Autodesk Inventor part; units mm, degrees
(part 2 of 2)
  line L664 (19.8841, -6.2623) -> (19.8841, -5.9623)
  arc A222 (19.8841, -6.2623) -> (19.8841, -7.2623) centre (19.8841, -6.7623) ccw
  arc A223 (18.2741, -5.9623) -> (18.2741, -7.5623) centre (18.2741, -6.7623) ccw
  arc A224 (18.2741, -5.9623) -> (18.2741, -7.5623) centre (18.2741, -6.7623) ccw
  line L665 (19.8841, -7.5623) -> (18.2741, -7.5623)
  line L666 (18.2741, -7.5623) -> (19.8841, -7.5623)
  line L667 (19.8841, -7.5623) -> (19.8841, -7.2623)
  circle A225 centre (18.2741, -6.7623) radius 0.5
  circle A226 centre (18.2741, -11.8423) radius 0.5
  circle A227 centre (6.8441, -19.2223) radius 0.5
  line L668 (-1.1159, -15.1823) -> (-1.1159, -16.1223)
  line L669 (-1.1159, -14.8823) -> (-1.1159, -16.4223)
  arc A228 (-1.1159, -17.4223) -> (-1.1159, -16.4223) centre (-1.1159, -16.9223) ccw
  circle A229 centre (0.4941, -16.9223) radius 0.5
  line L670 (-1.1159, -17.7223) -> (-1.1159, -18.6623)
  line L671 (-1.1159, -17.4223) -> (-1.1159, -18.9623)
  arc A230 (-1.1159, -19.9623) -> (-1.1159, -18.9623) centre (-1.1159, -19.4623) ccw
  line L672 (-1.1159, -20.2623) -> (-1.1159, -20.3323)
  arc A231 (7.3441, -20.8323) -> (6.3441, -20.8323) centre (6.8441, -20.8323) ccw
  line L673 (-1.1159, -19.9623) -> (-1.1159, -20.3323)
  arc A232 (19.8841, -8.8023) -> (19.8841, -9.8023) centre (19.8841, -9.3023) ccw
  arc A233 (19.8841, -13.8823) -> (19.8841, -14.8823) centre (19.8841, -14.3823) ccw
  arc A234 (19.8841, -18.9623) -> (19.8841, -19.9623) centre (19.8841, -19.4623) ccw
  line L674 (19.8841, -20.2623) -> (19.8841, -19.9623)
  circle A235 centre (18.2741, -19.4623) radius 0.5
  circle A236 centre (18.2741, -19.4623) radius 0.5
  circle A237 centre (9.3841, -19.2223) radius 0.5
  line L675 (-1.1159, -18.6623) -> (-1.1159, -18.9623)
  circle A238 centre (0.4941, -19.4623) radius 0.5
  circle A239 centre (0.4941, -19.4623) radius 0.5
  line L676 (-1.1159, -20.2623) -> (0.4941, -20.2623)
  line L677 (-1.1159, -19.9623) -> (-1.1159, -20.2623)
  arc A240 (-1.1159, -19.9623) -> (-1.1159, -18.9623) centre (-1.1159, -19.4623) ccw
  arc A241 (19.8841, -16.4223) -> (19.8841, -17.4223) centre (19.8841, -16.9223) ccw
  arc A242 (9.8841, -20.8323) -> (8.8841, -20.8323) centre (9.3841, -20.8323) ccw
  arc A243 (12.4241, -20.8323) -> (11.4241, -20.8323) centre (11.9241, -20.8323) ccw
  circle A244 centre (18.2741, -16.9223) radius 0.5
  circle A245 centre (18.2741, -14.3823) radius 0.5
  arc A246 (19.8841, -18.9623) -> (19.8841, -19.9623) centre (19.8841, -19.4623) ccw
  circle A247 centre (11.9241, -19.2223) radius 0.5
  line L678 (19.8841, -18.6623) -> (18.2741, -18.6623)
  line L679 (18.2741, -18.6623) -> (19.8841, -18.6623)
  arc A248 (18.2741, -18.6623) -> (18.2741, -20.2623) centre (18.2741, -19.4623) ccw
  arc A249 (18.2741, -18.6623) -> (18.2741, -20.2623) centre (18.2741, -19.4623) ccw
  line L680 (18.2741, -20.2623) -> (19.8841, -20.2623)
  line L681 (19.8841, -20.2623) -> (18.2741, -20.2623)
  line L682 (19.8841, -18.9623) -> (19.8841, -18.6623)
  arc A250 (0.4941, -20.2623) -> (0.4941, -18.6623) centre (0.4941, -19.4623) ccw
  arc A251 (0.4941, -20.2623) -> (0.4941, -18.6623) centre (0.4941, -19.4623) ccw
  line L683 (0.4941, -18.6623) -> (-1.1159, -18.6623)
  line L684 (-1.1159, -18.6623) -> (0.4941, -18.6623)
  line L685 (0.4941, -20.2623) -> (-1.1159, -20.2623)
  line L686 (-1.1159, -8.5023) -> (0.4941, -8.5023)
  line L687 (0.4941, -7.5623) -> (-1.1159, -7.5623)
  line L688 (-1.1159, -7.5623) -> (0.4941, -7.5623)
  line L689 (-1.1159, -7.2623) -> (-1.1159, -7.5623)
  circle A252 centre (0.4941, -6.7623) radius 0.5
  arc A253 (0.4941, -7.5623) -> (0.4941, -5.9623) centre (0.4941, -6.7623) ccw
  arc A254 (0.4941, -7.5623) -> (0.4941, -5.9623) centre (0.4941, -6.7623) ccw
  arc A255 (-1.1159, -7.2623) -> (-1.1159, -6.2623) centre (-1.1159, -6.7623) ccw
  line L690 (0.4941, -5.9623) -> (-1.1159, -5.9623)
  line L691 (-1.1159, -5.9623) -> (-1.1159, -6.2623)
  line L692 (-1.1159, -5.9623) -> (0.4941, -5.9623)
  line L693 (0.4941, -8.5023) -> (-1.1159, -8.5023)
  circle A256 centre (0.4941, -11.8423) radius 0.5
  arc A257 (-1.1159, -12.3423) -> (-1.1159, -11.3423) centre (-1.1159, -11.8423) ccw
  line L694 (-1.1159, -11.0423) -> (-1.1159, -11.3423)
  line L695 (-1.1159, -12.3423) -> (-1.1159, -12.6423)
  line L696 (-1.1159, -12.6423) -> (0.4941, -12.6423)
  line L697 (0.4941, -12.6423) -> (-1.1159, -12.6423)
  arc A258 (0.4941, -12.6423) -> (0.4941, -11.0423) centre (0.4941, -11.8423) ccw
  line L698 (-1.1159, -8.5023) -> (-1.1159, -8.8023)
  circle A259 centre (0.4941, -9.3023) radius 0.5
  arc A260 (-1.1159, -9.8023) -> (-1.1159, -8.8023) centre (-1.1159, -9.3023) ccw
  line L699 (-1.1159, -9.8023) -> (-1.1159, -10.1023)
  line L700 (-1.1159, -10.1023) -> (0.4941, -10.1023)
  line L701 (0.4941, -10.1023) -> (-1.1159, -10.1023)
  arc A261 (0.4941, -10.1023) -> (0.4941, -8.5023) centre (0.4941, -9.3023) ccw
  line L702 (0.4941, -11.0423) -> (-1.1159, -11.0423)
  line L703 (-1.1159, -11.0423) -> (0.4941, -11.0423)
  arc A262 (0.4941, -12.6423) -> (0.4941, -11.0423) centre (0.4941, -11.8423) ccw
  arc A263 (0.4941, -10.1023) -> (0.4941, -8.5023) centre (0.4941, -9.3023) ccw
  line L704 (-1.1159, -5.0223) -> (0.4941, -5.0223)
  line L705 (0.4941, -5.0223) -> (-1.1159, -5.0223)
  line L706 (-1.1159, -4.7223) -> (-1.1159, -5.0223)
  arc A264 (-1.1159, -4.7223) -> (-1.1159, -3.7223) centre (-1.1159, -4.2223) ccw
  line L707 (-1.1159, -3.4223) -> (-1.1159, -3.7223)
  line L708 (0.4941, -3.4223) -> (-1.1159, -3.4223)
  line L709 (-1.1159, -3.4223) -> (0.4941, -3.4223)
  circle A265 centre (0.4941, -4.2223) radius 0.5
  arc A266 (0.4941, -5.0223) -> (0.4941, -3.4223) centre (0.4941, -4.2223) ccw
  arc A267 (0.4941, -5.0223) -> (0.4941, -3.4223) centre (0.4941, -4.2223) ccw
  line L710 (18.2741, -3.4223) -> (19.8841, -3.4223)
  arc A268 (18.2741, -3.4223) -> (18.2741, -5.0223) centre (18.2741, -4.2223) ccw
  line L711 (19.8841, -5.0223) -> (18.2741, -5.0223)
  line L712 (18.2741, -5.0223) -> (19.8841, -5.0223)
  circle A269 centre (18.2741, -14.3823) radius 0.5
  arc A270 (18.2741, -3.4223) -> (18.2741, -5.0223) centre (18.2741, -4.2223) ccw
  circle A271 centre (18.2741, -11.8423) radius 0.5
  line L713 (19.8841, -11.0423) -> (18.2741, -11.0423)
  line L714 (18.2741, -11.0423) -> (19.8841, -11.0423)
  line L715 (19.8841, -11.3423) -> (19.8841, -11.0423)
  arc A272 (19.8841, -11.3423) -> (19.8841, -12.3423) centre (19.8841, -11.8423) ccw
  line L716 (18.2741, -12.6423) -> (19.8841, -12.6423)
  line L717 (19.8841, -12.6423) -> (18.2741, -12.6423)
  line L718 (19.8841, -12.6423) -> (19.8841, -12.3423)
  arc A273 (18.2741, -11.0423) -> (18.2741, -12.6423) centre (18.2741, -11.8423) ccw
  arc A274 (18.2741, -11.0423) -> (18.2741, -12.6423) centre (18.2741, -11.8423) ccw
  circle A275 centre (18.2741, -16.9223) radius 0.5
  line L719 (19.8841, -16.1223) -> (18.2741, -16.1223)
  line L720 (18.2741, -16.1223) -> (19.8841, -16.1223)
  line L721 (19.8841, -16.4223) -> (19.8841, -16.1223)
  arc A276 (19.8841, -16.4223) -> (19.8841, -17.4223) centre (19.8841, -16.9223) ccw
  arc A277 (18.2741, -16.1223) -> (18.2741, -17.7223) centre (18.2741, -16.9223) ccw
  arc A278 (18.2741, -16.1223) -> (18.2741, -17.7223) centre (18.2741, -16.9223) ccw
  line L722 (19.8841, -17.7223) -> (19.8841, -17.4223)
  line L723 (18.2741, -17.7223) -> (19.8841, -17.7223)
  line L724 (19.8841, -17.7223) -> (18.2741, -17.7223)
  circle A279 centre (11.9241, -19.2223) radius 0.5
  arc A280 (12.7241, -19.2223) -> (11.1241, -19.2223) centre (11.9241, -19.2223) ccw
  arc A281 (12.7241, -19.2223) -> (11.1241, -19.2223) centre (11.9241, -19.2223) ccw
  line L725 (12.7241, -20.8323) -> (12.7241, -19.2223)
  line L726 (12.7241, -19.2223) -> (12.7241, -20.8323)
  line L727 (12.4241, -20.8323) -> (12.7241, -20.8323)
  arc A282 (12.4241, -20.8323) -> (11.4241, -20.8323) centre (11.9241, -20.8323) ccw
  line L728 (11.1241, -20.8323) -> (11.4241, -20.8323)
  line L729 (11.1241, -20.8323) -> (11.1241, -19.2223)
  line L730 (11.1241, -19.2223) -> (11.1241, -20.8323)
  line L731 (-1.1159, -15.1823) -> (0.4941, -15.1823)
  circle A283 centre (6.8441, -19.2223) radius 0.5
  arc A284 (7.6441, -19.2223) -> (6.0441, -19.2223) centre (6.8441, -19.2223) ccw
  arc A285 (7.6441, -19.2223) -> (6.0441, -19.2223) centre (6.8441, -19.2223) ccw
  line L732 (7.6441, -20.8323) -> (7.6441, -19.2223)
  line L733 (7.6441, -19.2223) -> (7.6441, -20.8323)
  line L734 (7.3441, -20.8323) -> (7.6441, -20.8323)
  arc A286 (7.3441, -20.8323) -> (6.3441, -20.8323) centre (6.8441, -20.8323) ccw
  line L735 (6.0441, -19.2223) -> (6.0441, -20.8323)
  line L736 (6.0441, -20.8323) -> (6.0441, -19.2223)
  line L737 (6.0441, -20.8323) -> (6.3441, -20.8323)
  arc A287 (0.4941, -17.7223) -> (0.4941, -16.1223) centre (0.4941, -16.9223) ccw
  arc A288 (0.4941, -17.7223) -> (0.4941, -16.1223) centre (0.4941, -16.9223) ccw
  arc A289 (0.4941, -15.1823) -> (0.4941, -13.5823) centre (0.4941, -14.3823) ccw
  arc A290 (0.4941, -15.1823) -> (0.4941, -13.5823) centre (0.4941, -14.3823) ccw
  line L738 (0.4941, -13.5823) -> (-1.1159, -13.5823)
  line L739 (-1.1159, -13.5823) -> (0.4941, -13.5823)
  circle A291 centre (0.4941, -14.3823) radius 0.5
  line L740 (-1.1159, -13.5823) -> (-1.1159, -13.8823)
  arc A292 (-1.1159, -14.8823) -> (-1.1159, -13.8823) centre (-1.1159, -14.3823) ccw
  line L741 (-1.1159, -14.8823) -> (-1.1159, -15.1823)
  line L742 (0.4941, -15.1823) -> (-1.1159, -15.1823)
  circle A293 centre (0.4941, -16.9223) radius 0.5
  line L743 (-1.1159, -16.1223) -> (-1.1159, -16.4223)
  arc A294 (-1.1159, -17.4223) -> (-1.1159, -16.4223) centre (-1.1159, -16.9223) ccw
  line L744 (-1.1159, -17.7223) -> (0.4941, -17.7223)
  line L745 (-1.1159, -17.4223) -> (-1.1159, -17.7223)
  line L746 (-1.1159, -16.1223) -> (0.4941, -16.1223)
  line L747 (0.4941, -17.7223) -> (-1.1159, -17.7223)
  line L748 (0.4941, -16.1223) -> (-1.1159, -16.1223)
  line L749 (19.8841, 19.1377) -> (19.8841, 19.4377)
  arc A295 (19.8841, 19.1377) -> (19.8841, 18.1377) centre (19.8841, 18.6377) ccw
  line L750 (19.8841, 16.8977) -> (18.2741, 16.8977)
  line L751 (18.2741, 16.8977) -> (19.8841, 16.8977)
  line L752 (19.8841, 16.5977) -> (19.8841, 16.8977)
  circle A296 centre (18.2741, 16.0977) radius 0.5
  arc A297 (18.2741, 16.8977) -> (18.2741, 15.2977) centre (18.2741, 16.0977) ccw
  arc A298 (18.2741, 16.8977) -> (18.2741, 15.2977) centre (18.2741, 16.0977) ccw
  arc A299 (19.8841, 16.5977) -> (19.8841, 15.5977) centre (19.8841, 16.0977) ccw
  line L753 (18.2741, 15.2977) -> (19.8841, 15.2977)
  line L754 (19.8841, 15.2977) -> (18.2741, 15.2977)
  line L755 (19.8841, 15.2977) -> (19.8841, 15.5977)
  line L756 (13.0841, 31.4677) -> (13.0841, 26.4677)
  line L757 (13.0841, 31.4677) -> (13.0841, 26.4677)
  line L758 (12.7841, 31.4677) -> (12.7841, 26.4677)
  line L759 (12.9841, 30.8677) -> (12.9841, 31.4677)
  line L760 (12.7841, 26.4677) -> (13.0841, 26.4677)
  line L761 (13.3841, 30.8677) -> (12.9841, 30.8677)
  line L762 (12.7841, 31.4677) -> (13.0841, 31.4677)
  line L763 (12.9841, 31.4677) -> (13.3841, 31.4677)
  circle A300 centre (18.2741, 21.1777) radius 0.5
  arc A301 (19.8841, 21.6777) -> (19.8841, 20.6777) centre (19.8841, 21.1777) ccw
  line L764 (19.8841, 20.3777) -> (19.8841, 20.6777)
  line L765 (19.8841, 21.6777) -> (19.8841, 21.9777)
  line L766 (19.8841, 21.9777) -> (18.2741, 21.9777)
  line L767 (18.2741, 21.9777) -> (19.8841, 21.9777)
  line L768 (18.2741, 20.3777) -> (19.8841, 20.3777)
  line L769 (19.8841, 20.3777) -> (18.2741, 20.3777)
  arc A302 (18.2741, 21.9777) -> (18.2741, 20.3777) centre (18.2741, 21.1777) ccw
  arc A303 (18.2741, 21.9777) -> (18.2741, 20.3777) centre (18.2741, 21.1777) ccw
  line L770 (19.8841, 24.5177) -> (18.2741, 24.5177)
  line L771 (18.2741, 24.5177) -> (19.8841, 24.5177)
  line L772 (19.8841, 24.2177) -> (19.8841, 24.5177)
  arc A304 (18.2741, 24.5177) -> (18.2741, 22.9177) centre (18.2741, 23.7177) ccw
  arc A305 (18.2741, 24.5177) -> (18.2741, 22.9177) centre (18.2741, 23.7177) ccw
  circle A306 centre (18.2741, 23.7177) radius 0.5
  arc A307 (19.8841, 24.2177) -> (19.8841, 23.2177) centre (19.8841, 23.7177) ccw
  line L773 (18.2741, 22.9177) -> (19.8841, 22.9177)
  line L774 (19.8841, 22.9177) -> (18.2741, 22.9177)
  line L775 (19.8841, 22.9177) -> (19.8841, 23.2177)
  circle A308 centre (18.2741, 26.2577) radius 0.5
  arc A309 (19.8841, 26.7577) -> (19.8841, 25.7577) centre (19.8841, 26.2577) ccw
  line L776 (18.2741, 25.4577) -> (19.8841, 25.4577)
  line L777 (19.8841, 25.4577) -> (18.2741, 25.4577)
  line L778 (19.8841, 25.4577) -> (19.8841, 25.7577)
  line L779 (19.8841, 26.7577) -> (19.8841, 27.0577)
  arc A310 (18.2741, 27.0577) -> (18.2741, 25.4577) centre (18.2741, 26.2577) ccw
  arc A311 (18.2741, 27.0577) -> (18.2741, 25.4577) centre (18.2741, 26.2577) ccw
  line L780 (19.8841, 27.0577) -> (18.2741, 27.0577)
  line L781 (18.2741, 27.0577) -> (19.8841, 27.0577)
  circle A312 centre (18.2741, 28.7977) radius 0.5
  arc A313 (19.8841, 29.2977) -> (19.8841, 28.2977) centre (19.8841, 28.7977) ccw
  line L782 (19.8841, 27.9977) -> (19.8841, 28.2977)
  line L783 (19.8841, 29.2977) -> (19.8841, 29.5977)
  line L784 (19.8841, 29.5977) -> (18.2741, 29.5977)
  line L785 (18.2741, 29.5977) -> (19.8841, 29.5977)
  arc A314 (18.2741, 29.5977) -> (18.2741, 27.9977) centre (18.2741, 28.7977) ccw
  arc A315 (18.2741, 29.5977) -> (18.2741, 27.9977) centre (18.2741, 28.7977) ccw
  line L786 (18.2741, 27.9977) -> (19.8841, 27.9977)
  line L787 (19.8841, 27.9977) -> (18.2741, 27.9977)
  line L788 (13.3841, 31.4677) -> (13.3841, 30.8677)
  circle A316 centre (0.4941, 0.8577) radius 0.5
  arc A317 (-1.1159, 0.3577) -> (-1.1159, 1.3577) centre (-1.1159, 0.8577) ccw
  line L789 (-1.1159, 1.6577) -> (-1.1159, 1.3577)
  line L790 (-1.1159, 0.3577) -> (-1.1159, 0.0577)
  line L791 (-1.1159, 0.0577) -> (0.4941, 0.0577)
  arc A318 (0.4941, 0.0577) -> (0.4941, 1.6577) centre (0.4941, 0.8577) ccw
  arc A319 (0.4941, 0.0577) -> (0.4941, 1.6577) centre (0.4941, 0.8577) ccw
  line L792 (0.4941, 0.0577) -> (-1.1159, 0.0577)
  line L793 (0.4941, 1.6577) -> (-1.1159, 1.6577)
  line L794 (-1.1159, 1.6577) -> (0.4941, 1.6577)
  line L795 (-1.1159, 2.8977) -> (-1.1159, 2.5977)
  circle A320 centre (0.4941, 3.3977) radius 0.5
  arc A321 (-1.1159, 2.8977) -> (-1.1159, 3.8977) centre (-1.1159, 3.3977) ccw
  line L796 (-1.1159, 4.1977) -> (-1.1159, 3.8977)
  circle A322 centre (0.4941, 5.9377) radius 0.5
  arc A323 (-1.1159, 5.4377) -> (-1.1159, 6.4377) centre (-1.1159, 5.9377) ccw
  line L797 (-1.1159, 6.7377) -> (-1.1159, 6.4377)
  line L798 (-1.1159, 5.4377) -> (-1.1159, 5.1377)
  line L799 (-1.1159, 5.1377) -> (0.4941, 5.1377)
  line L800 (0.4941, 5.1377) -> (-1.1159, 5.1377)
  arc A324 (0.4941, 5.1377) -> (0.4941, 6.7377) centre (0.4941, 5.9377) ccw
  arc A325 (0.4941, 5.1377) -> (0.4941, 6.7377) centre (0.4941, 5.9377) ccw
  line L801 (0.4941, 6.7377) -> (-1.1159, 6.7377)
  line L802 (-1.1159, 6.7377) -> (0.4941, 6.7377)
  line L803 (-1.1159, 14.3577) -> (-1.1159, 14.0577)
  circle A326 centre (0.4941, 13.5577) radius 0.5
  line L804 (-1.1159, 13.0577) -> (-1.1159, 12.7577)
  line L805 (0.4941, 4.1977) -> (-1.1159, 4.1977)
  line L806 (-1.1159, 4.1977) -> (0.4941, 4.1977)
  line L807 (0.4941, 2.5977) -> (-1.1159, 2.5977)
  arc A327 (0.4941, 2.5977) -> (0.4941, 4.1977) centre (0.4941, 3.3977) ccw
  arc A328 (0.4941, 2.5977) -> (0.4941, 4.1977) centre (0.4941, 3.3977) ccw
  line L808 (-1.1159, 2.5977) -> (0.4941, 2.5977)
  arc A329 (-1.1159, 13.0577) -> (-1.1159, 14.0577) centre (-1.1159, 13.5577) ccw
  circle A330 centre (0.4941, 11.0177) radius 0.5
  arc A331 (-1.1159, 10.5177) -> (-1.1159, 11.5177) centre (-1.1159, 11.0177) ccw
  line L809 (-1.1159, 11.8177) -> (-1.1159, 11.5177)
  line L810 (-1.1159, 10.5177) -> (-1.1159, 10.2177)
  line L811 (-1.1159, 10.2177) -> (0.4941, 10.2177)
  line L812 (0.4941, 10.2177) -> (-1.1159, 10.2177)
  arc A332 (0.4941, 10.2177) -> (0.4941, 11.8177) centre (0.4941, 11.0177) ccw
  arc A333 (0.4941, 10.2177) -> (0.4941, 11.8177) centre (0.4941, 11.0177) ccw
  line L813 (-1.1159, 11.8177) -> (0.4941, 11.8177)
  line L814 (0.4941, 11.8177) -> (-1.1159, 11.8177)
  arc A334 (0.4941, 12.7577) -> (0.4941, 14.3577) centre (0.4941, 13.5577) ccw
  arc A335 (0.4941, 12.7577) -> (0.4941, 14.3577) centre (0.4941, 13.5577) ccw
  line L815 (0.4941, 14.3577) -> (-1.1159, 14.3577)
  line L816 (-1.1159, 14.3577) -> (0.4941, 14.3577)
  line L817 (0.4941, 12.7577) -> (-1.1159, 12.7577)
  line L818 (-1.1159, 12.7577) -> (0.4941, 12.7577)
  line L819 (19.8841, -3.4223) -> (18.2741, -3.4223)
  line L820 (19.8841, -3.7223) -> (19.8841, -3.4223)
  arc A336 (19.8841, -3.7223) -> (19.8841, -4.7223) centre (19.8841, -4.2223) ccw
  line L821 (19.8841, -5.0223) -> (19.8841, -4.7223)
  circle A337 centre (18.2741, -4.2223) radius 0.5
  arc A338 (19.8841, -13.8823) -> (19.8841, -14.8823) centre (19.8841, -14.3823) ccw
  line L822 (19.8841, -15.1823) -> (19.8841, -14.8823)
  line L823 (19.8841, -13.8823) -> (19.8841, -13.5823)
  line L824 (19.8841, -13.5823) -> (18.2741, -13.5823)
  line L825 (18.2741, -13.5823) -> (19.8841, -13.5823)
  circle A339 centre (9.3841, -19.2223) radius 0.5
  arc A340 (18.2741, -13.5823) -> (18.2741, -15.1823) centre (18.2741, -14.3823) ccw
  arc A341 (18.2741, -13.5823) -> (18.2741, -15.1823) centre (18.2741, -14.3823) ccw
  line L826 (18.2741, -15.1823) -> (19.8841, -15.1823)
  line L827 (19.8841, -15.1823) -> (18.2741, -15.1823)
  arc A342 (10.1841, -19.2223) -> (8.5841, -19.2223) centre (9.3841, -19.2223) ccw
  arc A343 (10.1841, -19.2223) -> (8.5841, -19.2223) centre (9.3841, -19.2223) ccw
  line L828 (8.5841, -19.2223) -> (8.5841, -20.8323)
  line L829 (8.5841, -20.8323) -> (8.5841, -19.2223)
  line L830 (10.1841, -20.8323) -> (10.1841, -19.2223)
  line L831 (10.1841, -19.2223) -> (10.1841, -20.8323)
  line L832 (9.8841, -20.8323) -> (10.1841, -20.8323)
  line L833 (8.5841, -20.8323) -> (8.8841, -20.8323)
  arc A344 (9.8841, -20.8323) -> (8.8841, -20.8323) centre (9.3841, -20.8323) ccw
  line L834 (57.2841, 13.4177) -> (56.4841, 13.4177)
  line L835 (56.4841, 13.4177) -> (57.2841, 13.4177)
  line L836 (57.2841, 13.4177) -> (57.2841, 13.9177)
  line L837 (57.2841, 13.9177) -> (56.4841, 13.9177)
  line L838 (57.2841, 13.9177) -> (57.2841, 13.4177)
  line L839 (56.4841, 13.9177) -> (57.2841, 13.9177)
  line L840 (56.4841, 13.9177) -> (56.4841, 13.4177)
  line L841 (56.4841, 13.4177) -> (56.4841, 13.9177)
  line L842 (56.4841, 8.9177) -> (57.2841, 8.9177)
  line L843 (56.4841, 8.4177) -> (56.4841, 8.9177)
  line L844 (57.2841, 8.4177) -> (56.4841, 8.4177)
  line L845 (57.2841, 8.9177) -> (57.2841, 8.4177)
  circle A345 centre (54.3841, 11.1677) radius 1.9
  circle A346 centre (54.3841, 11.1677) radius 1.9
  line L846 (57.2841, 8.9177) -> (56.4841, 8.9177)
  line L847 (56.4841, 8.9177) -> (56.4841, 8.4177)
  line L848 (57.2841, 8.4177) -> (57.2841, 8.9177)
  line L849 (56.4841, 8.4177) -> (57.2841, 8.4177)
  line L850 (52.2841, 8.9177) -> (52.2841, 8.4177)
  line L851 (52.2841, 8.4177) -> (51.4841, 8.4177)
  line L852 (51.4841, 8.4177) -> (51.4841, 8.9177)
  line L853 (51.4841, 8.9177) -> (52.2841, 8.9177)
  line L854 (52.2841, 8.9177) -> (51.4841, 8.9177)
  line L855 (52.2841, 8.4177) -> (52.2841, 8.9177)
  line L856 (51.4841, 8.9177) -> (51.4841, 8.4177)
  line L857 (51.4841, 8.4177) -> (52.2841, 8.4177)
  line L858 (52.2841, 13.4177) -> (51.4841, 13.4177)
  line L859 (51.4841, 13.4177) -> (51.4841, 13.9177)
  line L860 (51.4841, 13.9177) -> (52.2841, 13.9177)
  line L861 (52.2841, 13.4177) -> (52.2841, 13.9177)
  line L862 (52.2841, 13.9177) -> (52.2841, 13.4177)
  line L863 (52.2841, 13.9177) -> (51.4841, 13.9177)
  line L864 (51.4841, 13.9177) -> (51.4841, 13.4177)
  line L865 (51.4841, 13.4177) -> (52.2841, 13.4177)
  arc A347 (59.9841, 13.3217) -> (59.9841, 9.0136) centre (54.3841, 11.1677) ccw
  line L866 (59.9841, 9.0136) -> (59.9841, 13.3217)
  circle A348 centre (54.3841, 11.1677) radius 4.5
  circle A349 centre (54.3841, 11.1677) radius 4.5
  line L867 (59.9841, 9.0136) -> (59.9841, 13.3217)
  arc A350 (59.9841, 13.3217) -> (59.9841, 9.0136) centre (54.3841, 11.1677) ccw
  line L868 (66.6341, 18.2677) -> (66.6341, 19.0677)
  line L869 (66.6341, 19.0677) -> (66.6341, 18.2677)
  line L870 (66.6341, 18.2677) -> (67.1341, 18.2677)
  line L871 (67.1341, 18.2677) -> (67.1341, 19.0677)
  line L872 (67.1341, 18.2677) -> (66.6341, 18.2677)
  line L873 (67.1341, 19.0677) -> (67.1341, 18.2677)
  line L874 (67.1341, 19.0677) -> (66.6341, 19.0677)
  line L875 (66.6341, 19.0677) -> (67.1341, 19.0677)
  line L876 (62.1341, 19.0677) -> (62.1341, 18.2677)
  line L877 (61.6341, 19.0677) -> (62.1341, 19.0677)
  line L878 (61.6341, 18.2677) -> (61.6341, 19.0677)
  line L879 (62.1341, 18.2677) -> (61.6341, 18.2677)
  circle A351 centre (64.3841, 21.1677) radius 1.9
  circle A352 centre (64.3841, 21.1677) radius 1.9
  line L880 (62.1341, 18.2677) -> (62.1341, 19.0677)
  line L881 (62.1341, 19.0677) -> (61.6341, 19.0677)
  line L882 (61.6341, 18.2677) -> (62.1341, 18.2677)
  line L883 (61.6341, 19.0677) -> (61.6341, 18.2677)
  line L884 (62.1341, 23.2677) -> (61.6341, 23.2677)
  line L885 (61.6341, 23.2677) -> (61.6341, 24.0677)
  line L886 (61.6341, 24.0677) -> (62.1341, 24.0677)
  line L887 (62.1341, 24.0677) -> (62.1341, 23.2677)
  line L888 (62.1341, 23.2677) -> (62.1341, 24.0677)
  line L889 (61.6341, 23.2677) -> (62.1341, 23.2677)
  line L890 (62.1341, 24.0677) -> (61.6341, 24.0677)
  line L891 (61.6341, 24.0677) -> (61.6341, 23.2677)
  line L892 (66.6341, 23.2677) -> (66.6341, 24.0677)
  line L893 (66.6341, 24.0677) -> (67.1341, 24.0677)
  line L894 (67.1341, 24.0677) -> (67.1341, 23.2677)
  line L895 (66.6341, 23.2677) -> (67.1341, 23.2677)
  line L896 (67.1341, 23.2677) -> (66.6341, 23.2677)
  line L897 (67.1341, 23.2677) -> (67.1341, 24.0677)
  line L898 (67.1341, 24.0677) -> (66.6341, 24.0677)
  line L899 (66.6341, 24.0677) -> (66.6341, 23.2677)
  arc A353 (66.5382, 15.5677) -> (62.2301, 15.5677) centre (64.3841, 21.1677) ccw
  line L900 (62.2301, 15.5677) -> (66.5382, 15.5677)
  circle A354 centre (64.3841, 21.1677) radius 4.5
  circle A355 centre (64.3841, 21.1677) radius 4.5
  line L901 (62.2301, 15.5677) -> (66.5382, 15.5677)
  arc A356 (66.5382, 15.5677) -> (62.2301, 15.5677) centre (64.3841, 21.1677) ccw
  line L902 (62.1341, 4.0677) -> (62.1341, 3.2677)
  line L903 (62.1341, 3.2677) -> (62.1341, 4.0677)
  line L904 (62.1341, 4.0677) -> (61.6341, 4.0677)
  line L905 (61.6341, 4.0677) -> (61.6341, 3.2677)
  line L906 (61.6341, 4.0677) -> (62.1341, 4.0677)
  line L907 (61.6341, 3.2677) -> (61.6341, 4.0677)
  line L908 (61.6341, 3.2677) -> (62.1341, 3.2677)
  line L909 (62.1341, 3.2677) -> (61.6341, 3.2677)
  line L910 (66.6341, 3.2677) -> (66.6341, 4.0677)
  line L911 (67.1341, 3.2677) -> (66.6341, 3.2677)
  line L912 (67.1341, 4.0677) -> (67.1341, 3.2677)
  line L913 (66.6341, 4.0677) -> (67.1341, 4.0677)
  circle A357 centre (64.3841, 1.1677) radius 1.9
  circle A358 centre (64.3841, 1.1677) radius 1.9
  line L914 (66.6341, 4.0677) -> (66.6341, 3.2677)
  line L915 (66.6341, 3.2677) -> (67.1341, 3.2677)
  line L916 (67.1341, 4.0677) -> (66.6341, 4.0677)
  line L917 (67.1341, 3.2677) -> (67.1341, 4.0677)
  line L918 (66.6341, -0.9323) -> (67.1341, -0.9323)
  line L919 (67.1341, -0.9323) -> (67.1341, -1.7323)
  line L920 (67.1341, -1.7323) -> (66.6341, -1.7323)
  line L921 (66.6341, -1.7323) -> (66.6341, -0.9323)
  line L922 (66.6341, -0.9323) -> (66.6341, -1.7323)
  line L923 (67.1341, -0.9323) -> (66.6341, -0.9323)
  line L924 (66.6341, -1.7323) -> (67.1341, -1.7323)
  line L925 (67.1341, -1.7323) -> (67.1341, -0.9323)
  line L926 (62.1341, -0.9323) -> (62.1341, -1.7323)
  line L927 (62.1341, -1.7323) -> (61.6341, -1.7323)
  line L928 (61.6341, -1.7323) -> (61.6341, -0.9323)
  line L929 (62.1341, -0.9323) -> (61.6341, -0.9323)
  line L930 (61.6341, -0.9323) -> (62.1341, -0.9323)
  line L931 (61.6341, -0.9323) -> (61.6341, -1.7323)
  line L932 (61.6341, -1.7323) -> (62.1341, -1.7323)
  line L933 (62.1341, -1.7323) -> (62.1341, -0.9323)
  arc A359 (62.2301, 6.7677) -> (66.5382, 6.7677) centre (64.3841, 1.1677) ccw
  line L934 (66.5382, 6.7677) -> (62.2301, 6.7677)
  circle A360 centre (64.3841, 1.1677) radius 4.5
  circle A361 centre (64.3841, 1.1677) radius 4.5
  line L935 (66.5382, 6.7677) -> (62.2301, 6.7677)
  arc A362 (62.2301, 6.7677) -> (66.5382, 6.7677) centre (64.3841, 1.1677) ccw
  line L936 (71.4841, 8.9177) -> (72.2841, 8.9177)
  line L937 (72.2841, 8.9177) -> (71.4841, 8.9177)
  line L938 (71.4841, 8.9177) -> (71.4841, 8.4177)
  line L939 (71.4841, 8.4177) -> (72.2841, 8.4177)
  line L940 (71.4841, 8.4177) -> (71.4841, 8.9177)
  line L941 (72.2841, 8.4177) -> (71.4841, 8.4177)
  line L942 (72.2841, 8.4177) -> (72.2841, 8.9177)
  line L943 (72.2841, 8.9177) -> (72.2841, 8.4177)
  line L944 (72.2841, 13.4177) -> (71.4841, 13.4177)
  line L945 (72.2841, 13.9177) -> (72.2841, 13.4177)
  line L946 (71.4841, 13.9177) -> (72.2841, 13.9177)
  line L947 (71.4841, 13.4177) -> (71.4841, 13.9177)
  circle A363 centre (74.3841, 11.1677) radius 1.9
  circle A364 centre (74.3841, 11.1677) radius 1.9
  line L948 (71.4841, 13.4177) -> (72.2841, 13.4177)
  line L949 (72.2841, 13.4177) -> (72.2841, 13.9177)
  line L950 (71.4841, 13.9177) -> (71.4841, 13.4177)
  line L951 (72.2841, 13.9177) -> (71.4841, 13.9177)
  line L952 (76.4841, 13.4177) -> (76.4841, 13.9177)
  line L953 (76.4841, 13.9177) -> (77.2841, 13.9177)
  line L954 (77.2841, 13.9177) -> (77.2841, 13.4177)
  line L955 (77.2841, 13.4177) -> (76.4841, 13.4177)
  line L956 (76.4841, 13.4177) -> (77.2841, 13.4177)
  line L957 (76.4841, 13.9177) -> (76.4841, 13.4177)
  line L958 (77.2841, 13.4177) -> (77.2841, 13.9177)
  line L959 (77.2841, 13.9177) -> (76.4841, 13.9177)
  line L960 (76.4841, 8.9177) -> (77.2841, 8.9177)
  line L961 (77.2841, 8.9177) -> (77.2841, 8.4177)
  line L962 (77.2841, 8.4177) -> (76.4841, 8.4177)
  line L963 (76.4841, 8.9177) -> (76.4841, 8.4177)
  line L964 (76.4841, 8.4177) -> (76.4841, 8.9177)
  line L965 (76.4841, 8.4177) -> (77.2841, 8.4177)
  line L966 (77.2841, 8.4177) -> (77.2841, 8.9177)
  line L967 (77.2841, 8.9177) -> (76.4841, 8.9177)
  arc A365 (68.7841, 9.0136) -> (68.7841, 13.3217) centre (74.3841, 11.1677) ccw
  line L968 (68.7841, 13.3217) -> (68.7841, 9.0136)
  circle A366 centre (74.3841, 11.1677) radius 4.5
  circle A367 centre (74.3841, 11.1677) radius 4.5
  line L969 (68.7841, 13.3217) -> (68.7841, 9.0136)
  arc A368 (68.7841, 9.0136) -> (68.7841, 13.3217) centre (74.3841, 11.1677) ccw
  line L970 (-43.3659, 18.2677) -> (-43.3659, 19.0677)
  line L971 (-43.3659, 19.0677) -> (-43.3659, 18.2677)
  line L972 (-43.3659, 18.2677) -> (-42.8659, 18.2677)
  line L973 (-42.8659, 18.2677) -> (-42.8659, 19.0677)
  line L974 (-42.8659, 18.2677) -> (-43.3659, 18.2677)
  line L975 (-42.8659, 19.0677) -> (-42.8659, 18.2677)
  line L976 (-42.8659, 19.0677) -> (-43.3659, 19.0677)
  line L977 (-43.3659, 19.0677) -> (-42.8659, 19.0677)
  line L978 (-47.8659, 19.0677) -> (-47.8659, 18.2677)
  line L979 (-48.3659, 19.0677) -> (-47.8659, 19.0677)
  line L980 (-48.3659, 18.2677) -> (-48.3659, 19.0677)
  line L981 (-47.8659, 18.2677) -> (-48.3659, 18.2677)
  circle A369 centre (-45.6159, 21.1677) radius 1.9
  circle A370 centre (-45.6159, 21.1677) radius 1.9
  line L982 (-47.8659, 18.2677) -> (-47.8659, 19.0677)
  line L983 (-47.8659, 19.0677) -> (-48.3659, 19.0677)
  line L984 (-48.3659, 18.2677) -> (-47.8659, 18.2677)
  line L985 (-48.3659, 19.0677) -> (-48.3659, 18.2677)
  line L986 (-47.8659, 23.2677) -> (-48.3659, 23.2677)
  line L987 (-48.3659, 23.2677) -> (-48.3659, 24.0677)
  line L988 (-48.3659, 24.0677) -> (-47.8659, 24.0677)
  line L989 (-47.8659, 24.0677) -> (-47.8659, 23.2677)
  line L990 (-47.8659, 23.2677) -> (-47.8659, 24.0677)
  line L991 (-48.3659, 23.2677) -> (-47.8659, 23.2677)
  line L992 (-47.8659, 24.0677) -> (-48.3659, 24.0677)
  line L993 (-48.3659, 24.0677) -> (-48.3659, 23.2677)
  line L994 (-43.3659, 23.2677) -> (-43.3659, 24.0677)
  line L995 (-43.3659, 24.0677) -> (-42.8659, 24.0677)
  line L996 (-42.8659, 24.0677) -> (-42.8659, 23.2677)
  line L997 (-43.3659, 23.2677) -> (-42.8659, 23.2677)
  line L998 (-42.8659, 23.2677) -> (-43.3659, 23.2677)
  line L999 (-42.8659, 23.2677) -> (-42.8659, 24.0677)
  line L1000 (-42.8659, 24.0677) -> (-43.3659, 24.0677)
  line L1001 (-43.3659, 24.0677) -> (-43.3659, 23.2677)
  line L1002 (-47.7699, 15.5677) -> (-43.4618, 15.5677)
  circle A371 centre (-45.6159, 21.1677) radius 4.5
  circle A372 centre (-45.6159, 21.1677) radius 4.5
  line L1003 (-47.7699, 15.5677) -> (-43.4618, 15.5677)
  arc A373 (-43.4618, 15.5677) -> (-47.7699, 15.5677) centre (-45.6159, 21.1677) ccw
  line L1004 (-47.8659, 4.0677) -> (-47.8659, 3.2677)
  line L1005 (-47.8659, 3.2677) -> (-47.8659, 4.0677)
  line L1006 (-47.8659, 4.0677) -> (-48.3659, 4.0677)
  line L1007 (-48.3659, 4.0677) -> (-48.3659, 3.2677)
  line L1008 (-48.3659, 4.0677) -> (-47.8659, 4.0677)
  line L1009 (-48.3659, 3.2677) -> (-48.3659, 4.0677)
  line L1010 (-48.3659, 3.2677) -> (-47.8659, 3.2677)
  line L1011 (-47.8659, 3.2677) -> (-48.3659, 3.2677)
  line L1012 (-43.3659, 3.2677) -> (-43.3659, 4.0677)
  line L1013 (-42.8659, 3.2677) -> (-43.3659, 3.2677)
  line L1014 (-42.8659, 4.0677) -> (-42.8659, 3.2677)
  line L1015 (-43.3659, 4.0677) -> (-42.8659, 4.0677)
  circle A374 centre (-45.6159, 1.1677) radius 1.9
  circle A375 centre (-45.6159, 1.1677) radius 1.9
  line L1016 (-43.3659, 4.0677) -> (-43.3659, 3.2677)
  line L1017 (-43.3659, 3.2677) -> (-42.8659, 3.2677)
  line L1018 (-42.8659, 4.0677) -> (-43.3659, 4.0677)
  line L1019 (-42.8659, 3.2677) -> (-42.8659, 4.0677)
  line L1020 (-43.3659, -0.9323) -> (-42.8659, -0.9323)
  line L1021 (-42.8659, -0.9323) -> (-42.8659, -1.7323)
  line L1022 (-42.8659, -1.7323) -> (-43.3659, -1.7323)
  line L1023 (-43.3659, -1.7323) -> (-43.3659, -0.9323)
  line L1024 (-43.3659, -0.9323) -> (-43.3659, -1.7323)
  line L1025 (-42.8659, -0.9323) -> (-43.3659, -0.9323)
  line L1026 (-43.3659, -1.7323) -> (-42.8659, -1.7323)
  line L1027 (-42.8659, -1.7323) -> (-42.8659, -0.9323)
  line L1028 (-47.8659, -0.9323) -> (-47.8659, -1.7323)
  line L1029 (-47.8659, -1.7323) -> (-48.3659, -1.7323)
  line L1030 (-48.3659, -1.7323) -> (-48.3659, -0.9323)
  line L1031 (-47.8659, -0.9323) -> (-48.3659, -0.9323)
  line L1032 (-48.3659, -0.9323) -> (-47.8659, -0.9323)
  line L1033 (-48.3659, -0.9323) -> (-48.3659, -1.7323)
  line L1034 (-48.3659, -1.7323) -> (-47.8659, -1.7323)
  line L1035 (-47.8659, -1.7323) -> (-47.8659, -0.9323)
  arc A376 (-47.7699, 6.7677) -> (-43.4618, 6.7677) centre (-45.6159, 1.1677) ccw
  line L1036 (-43.4618, 6.7677) -> (-47.7699, 6.7677)
  circle A377 centre (-45.6159, 1.1677) radius 4.5
  circle A378 centre (-45.6159, 1.1677) radius 4.5
  line L1037 (-43.4618, 6.7677) -> (-47.7699, 6.7677)
  arc A379 (-47.7699, 6.7677) -> (-43.4618, 6.7677) centre (-45.6159, 1.1677) ccw
  line L1038 (-38.5159, 8.9177) -> (-37.7159, 8.9177)
  line L1039 (-37.7159, 8.9177) -> (-38.5159, 8.9177)
  line L1040 (-38.5159, 8.9177) -> (-38.5159, 8.4177)
  line L1041 (-38.5159, 8.4177) -> (-37.7159, 8.4177)
  line L1042 (-38.5159, 8.4177) -> (-38.5159, 8.9177)
  line L1043 (-37.7159, 8.4177) -> (-38.5159, 8.4177)
  line L1044 (-37.7159, 8.4177) -> (-37.7159, 8.9177)
  line L1045 (-37.7159, 8.9177) -> (-37.7159, 8.4177)
  line L1046 (-37.7159, 13.4177) -> (-38.5159, 13.4177)
  line L1047 (-37.7159, 13.9177) -> (-37.7159, 13.4177)
  line L1048 (-38.5159, 13.9177) -> (-37.7159, 13.9177)
  line L1049 (-38.5159, 13.4177) -> (-38.5159, 13.9177)
  circle A380 centre (-35.6159, 11.1677) radius 1.9
  circle A381 centre (-35.6159, 11.1677) radius 1.9
  line L1050 (-38.5159, 13.4177) -> (-37.7159, 13.4177)
  line L1051 (-37.7159, 13.4177) -> (-37.7159, 13.9177)
  line L1052 (-38.5159, 13.9177) -> (-38.5159, 13.4177)
  line L1053 (-37.7159, 13.9177) -> (-38.5159, 13.9177)
  line L1054 (-33.5159, 13.4177) -> (-33.5159, 13.9177)
  line L1055 (-33.5159, 13.9177) -> (-32.7159, 13.9177)
  line L1056 (-32.7159, 13.9177) -> (-32.7159, 13.4177)
  line L1057 (-32.7159, 13.4177) -> (-33.5159, 13.4177)
  line L1058 (-33.5159, 13.4177) -> (-32.7159, 13.4177)
  line L1059 (-33.5159, 13.9177) -> (-33.5159, 13.4177)
  line L1060 (-32.7159, 13.4177) -> (-32.7159, 13.9177)
  line L1061 (-32.7159, 13.9177) -> (-33.5159, 13.9177)
  line L1062 (-33.5159, 8.9177) -> (-32.7159, 8.9177)
  line L1063 (-32.7159, 8.9177) -> (-32.7159, 8.4177)
  line L1064 (-32.7159, 8.4177) -> (-33.5159, 8.4177)
  line L1065 (-33.5159, 8.9177) -> (-33.5159, 8.4177)
  line L1066 (-33.5159, 8.4177) -> (-33.5159, 8.9177)
  line L1067 (-33.5159, 8.4177) -> (-32.7159, 8.4177)
  line L1068 (-32.7159, 8.4177) -> (-32.7159, 8.9177)
  line L1069 (-32.7159, 8.9177) -> (-33.5159, 8.9177)
  arc A382 (-41.2159, 9.0136) -> (-41.2159, 13.3217) centre (-35.6159, 11.1677) ccw
  line L1070 (-41.2159, 13.3217) -> (-41.2159, 9.0136)
  circle A383 centre (-35.6159, 11.1677) radius 4.5
  circle A384 centre (-35.6159, 11.1677) radius 4.5
  line L1071 (-41.2159, 13.3217) -> (-41.2159, 9.0136)
  arc A385 (-41.2159, 9.0136) -> (-41.2159, 13.3217) centre (-35.6159, 11.1677) ccw
  line L1072 (-52.7159, 13.4177) -> (-53.5159, 13.4177)
  line L1073 (-53.5159, 13.4177) -> (-52.7159, 13.4177)
  line L1074 (-52.7159, 13.4177) -> (-52.7159, 13.9177)
  line L1075 (-52.7159, 13.9177) -> (-53.5159, 13.9177)
  line L1076 (-52.7159, 13.9177) -> (-52.7159, 13.4177)
  line L1077 (-53.5159, 13.9177) -> (-52.7159, 13.9177)
  line L1078 (-53.5159, 13.9177) -> (-53.5159, 13.4177)
  line L1079 (-53.5159, 13.4177) -> (-53.5159, 13.9177)
  line L1080 (-53.5159, 8.9177) -> (-52.7159, 8.9177)
  line L1081 (-53.5159, 8.4177) -> (-53.5159, 8.9177)
  line L1082 (-52.7159, 8.4177) -> (-53.5159, 8.4177)
  line L1083 (-52.7159, 8.9177) -> (-52.7159, 8.4177)
  circle A386 centre (-55.6159, 11.1677) radius 1.9
  circle A387 centre (-55.6159, 11.1677) radius 1.9
  line L1084 (-52.7159, 8.9177) -> (-53.5159, 8.9177)
  line L1085 (-53.5159, 8.9177) -> (-53.5159, 8.4177)
  line L1086 (-52.7159, 8.4177) -> (-52.7159, 8.9177)
  line L1087 (-53.5159, 8.4177) -> (-52.7159, 8.4177)
  line L1088 (-57.7159, 8.9177) -> (-57.7159, 8.4177)
  line L1089 (-57.7159, 8.4177) -> (-58.5159, 8.4177)
  line L1090 (-58.5159, 8.4177) -> (-58.5159, 8.9177)
  line L1091 (-58.5159, 8.9177) -> (-57.7159, 8.9177)
  line L1092 (-57.7159, 8.9177) -> (-58.5159, 8.9177)
  line L1093 (-57.7159, 8.4177) -> (-57.7159, 8.9177)
  line L1094 (-58.5159, 8.9177) -> (-58.5159, 8.4177)
  line L1095 (-58.5159, 8.4177) -> (-57.7159, 8.4177)
  line L1096 (-57.7159, 13.4177) -> (-58.5159, 13.4177)
  line L1097 (-58.5159, 13.4177) -> (-58.5159, 13.9177)
  line L1098 (-58.5159, 13.9177) -> (-57.7159, 13.9177)
  line L1099 (-57.7159, 13.4177) -> (-57.7159, 13.9177)
  line L1100 (-57.7159, 13.9177) -> (-57.7159, 13.4177)
  line L1101 (-57.7159, 13.9177) -> (-58.5159, 13.9177)
  line L1102 (-58.5159, 13.9177) -> (-58.5159, 13.4177)
  line L1103 (-58.5159, 13.4177) -> (-57.7159, 13.4177)
  arc A388 (-50.0159, 13.3217) -> (-50.0159, 9.0136) centre (-55.6159, 11.1677) ccw
  line L1104 (-50.0159, 9.0136) -> (-50.0159, 13.3217)
  circle A389 centre (-55.6159, 11.1677) radius 4.5
  circle A390 centre (-55.6159, 11.1677) radius 4.5
  line L1105 (-50.0159, 9.0136) -> (-50.0159, 13.3217)
  arc A391 (-50.0159, 13.3217) -> (-50.0159, 9.0136) centre (-55.6159, 11.1677) ccw
  point P0 (37.3841, -10.6323)
  point P1 (-18.6159, -10.6323)
  dimension "d2" = 150
  constraints: 2204 end point, 392 centre point, 392 point on circle, 6 other
  measures "d2" distance of L2.start L36.start
sketch "Náčrt2" plane through (0, 0, 0) normal (0, 0, 1) x (1, 0, 0)
  line L0 (-66.6159, 31.6677) -> (85.3841, 31.6677)
  line L1 (85.3841, 31.6677) -> (85.3841, -29.3323)
  line L2 (85.3841, -29.3323) -> (-66.6159, -29.3323)
  line L3 (-66.6159, -29.3323) -> (-66.6159, 31.6677)
  line L4 (84.3841, 31.1677) -> (-65.6159, 31.1677) projected
  line L5 (-65.6159, 31.1677) -> (-65.6159, -28.8323) projected
  line L6 (-65.6159, -28.8323) -> (84.3841, -28.8323) projected
  line L7 (84.3841, -28.8323) -> (84.3841, 31.1677) projected
  arc A0 (-43.4618, 15.5677) -> (-47.7699, 15.5677) centre (-45.6159, 21.1677) ccw projected
  line L8 (-47.7699, 15.5677) -> (-43.4618, 15.5677) projected
  line L9 (-50.0159, 9.0136) -> (-50.0159, 13.3217) projected
  arc A1 (-50.0159, 13.3217) -> (-50.0159, 9.0136) centre (-55.6159, 11.1677) ccw projected
  line L10 (-43.4618, 6.7677) -> (-47.7699, 6.7677) projected
  arc A2 (-47.7699, 6.7677) -> (-43.4618, 6.7677) centre (-45.6159, 1.1677) ccw projected
  line L11 (-41.2159, 13.3217) -> (-41.2159, 9.0136) projected
  arc A3 (-41.2159, 9.0136) -> (-41.2159, 13.3217) centre (-35.6159, 11.1677) ccw projected
  circle A4 centre (-18.6159, -10.6323) radius 12 projected
  circle A5 centre (37.3841, -10.6323) radius 12 projected
  arc A6 (59.9841, 13.3217) -> (59.9841, 9.0136) centre (54.3841, 11.1677) ccw projected
  line L12 (59.9841, 9.0136) -> (59.9841, 13.3217) projected
  arc A7 (66.5382, 15.5677) -> (62.2301, 15.5677) centre (64.3841, 21.1677) ccw projected
  line L13 (62.2301, 15.5677) -> (66.5382, 15.5677) projected
  line L14 (68.7841, 13.3217) -> (68.7841, 9.0136) projected
  arc A8 (68.7841, 9.0136) -> (68.7841, 13.3217) centre (74.3841, 11.1677) ccw projected
  line L15 (66.5382, 6.7677) -> (62.2301, 6.7677) projected
  arc A9 (62.2301, 6.7677) -> (66.5382, 6.7677) centre (64.3841, 1.1677) ccw projected
  point P0 (0, 0)
  dimension "d5" = 0.5
  dimension "d6" = 0.5
  dimension "d7" = 1
  dimension "d8" = 1
  constraints: 8 end point, 2 parallel, 1 horizontal, 1 perpendicular
  measures "d5" distance between parallel lines of L4 L0
  measures "d6" distance between parallel lines of L6 L2
  measures "d7" distance between parallel lines of L5 L3
  measures "d8" distance between parallel lines of L7 L1
extrude "Vysunutí1" add sketch "Náčrt2" along normal blind 10 contours L0 L1 L2 L3 | L7 L6 L5 L4 | L8 A0 | A1 L9 | A2 L10 | A3 L11 | A4 | A5 | L12 A6 | L13 A7 | A8 L14 | A9 L15
sketch "Náčrt3" plane through (0, 0, 0) normal (0, 0, -1) x (-1, 0, 0)
  arc A0 (-62.2301, 15.5677) -> (-66.5382, 15.5677) centre (-64.3841, 21.1677) ccw projected
  line L0 (-62.2301, 15.5677) -> (-66.5382, 15.5677) projected
  arc A1 (-68.7841, 13.3217) -> (-68.7841, 9.0136) centre (-74.3841, 11.1677) ccw projected
  line L1 (-68.7841, 13.3217) -> (-68.7841, 9.0136) projected
  line L2 (-66.5382, 6.7677) -> (-62.2301, 6.7677) projected
  arc A2 (-66.5382, 6.7677) -> (-62.2301, 6.7677) centre (-64.3841, 1.1677) ccw projected
  line L3 (-59.9841, 9.0136) -> (-59.9841, 13.3217) projected
  arc A3 (-59.9841, 9.0136) -> (-59.9841, 13.3217) centre (-54.3841, 11.1677) ccw projected
  circle A4 centre (-37.3841, -10.6323) radius 12 projected
  circle A5 centre (18.6159, -10.6323) radius 12 projected
  arc A6 (41.2159, 13.3217) -> (41.2159, 9.0136) centre (35.6159, 11.1677) ccw projected
  line L4 (41.2159, 13.3217) -> (41.2159, 9.0136) projected
  arc A7 (47.7699, 15.5677) -> (43.4618, 15.5677) centre (45.6159, 21.1677) ccw projected
  line L5 (47.7699, 15.5677) -> (43.4618, 15.5677) projected
  arc A8 (50.0159, 9.0136) -> (50.0159, 13.3217) centre (55.6159, 11.1677) ccw projected
  line L6 (50.0159, 9.0136) -> (50.0159, 13.3217) projected
  line L7 (43.4618, 6.7677) -> (47.7699, 6.7677) projected
  arc A9 (43.4618, 6.7677) -> (47.7699, 6.7677) centre (45.6159, 1.1677) ccw projected
  point P0 (0, 0)
extrude "Vysunutí2" cut sketch "Náčrt3" against normal through all
sketch "Náčrt4" plane through (0, 0, 0) normal (0, 0, -1) x (-1, 0, 0)
  line L0 (-85.3841, -29.3323) -> (-85.3841, 31.6677) projected
  line L1 (66.6159, 31.6677) -> (66.6159, -29.3323) projected
  line L2 (-85.3841, 31.6677) -> (66.6159, 31.6677) projected
  line L3 (66.6159, -29.3323) -> (-85.3841, -29.3323) projected
  circle A0 centre (-9.3841, 19.2804) radius 3.5
  point P0 (0, 0)
  dimension "d13" = 76
  dimension "d14" = 76
  dimension "d15" = 7
  constraints: 1 centre point, 1 coincident
  measures "d13" distance from line of L0 point (-9.384, 19.28)
  measures "d14" distance from line of L1 point (-9.384, 19.28)
  measures "d15" diameter of A0
extrude "Vysunutí3" cut sketch "Náčrt4" against normal through all contours A0
